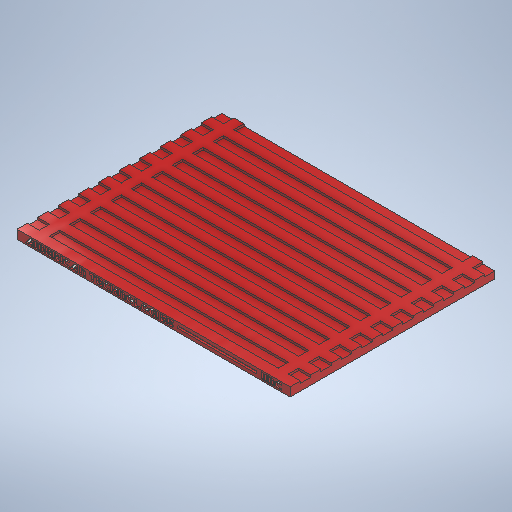
# Autodesk Inventor part: AT-IMC lid
Saved by Autodesk Inventor 2025 (Build 290162000, 162)
## iProperties
Created: 2025-05-10
Part Number: AT-IMC lid
Material: Generic
Document SubType Name: Modeling
Designer: thesn
Density: 1 g/cm^3
Appearance: Default
Author: thesn
Autodesk Inventor part; units mm, degrees
ref_plane "YZ Plane" through (0, 0, 0) normal (1, 0, 0) x (0, 1, 0)
ref_plane "XZ Plane" through (0, 0, 0) normal (0, 1, 0) x (-1, 0, 0)
ref_plane "XY Plane" through (0, 0, 0) normal (0, 0, 1) x (1, 0, 0)
sketch "Sketch1" plane through (0, 0, 0) normal (0, 0, 1) x (1, 0, 0)
  line L0 (0, 0) -> (203.2, 0)
  line L1 (203.2, 0) -> (203.2, 5.08)
  line L2 (203.2, 5.08) -> (0, 5.08)
  line L3 (0, 5.08) -> (0, 0)
  dimension "d0" = 203.2
  dimension "d1" = 5.08
  constraints: 8 end point, 2 parallel, 1 horizontal, 1 perpendicular
  measures "d0" distance of L2.end L1.end
  measures "d1" distance of L1.end L0.end
extrude "Extrusion1" add sketch "Sketch1" along normal blind 152.4
sketch "Sketch2" plane through (0, 0, 0) normal (0, -1, 0) x (1, 0, 0)
  line L0 (5.08, 147.32) -> (198.12, 147.32)
  line L1 (198.12, 147.32) -> (198.12, 5.08)
  line L2 (198.12, 5.08) -> (5.08, 5.08)
  line L3 (5.08, 5.08) -> (5.08, 147.32)
  line L4 (0, 152.4) -> (203.2, 152.4) projected
  line L5 (203.2, 0) -> (203.2, 152.4) projected
  point P0 (0, 0)
  point P1 (101.6, 152.4)
  point P2 (101.6, 147.32)
  point P3 (203.2, 76.2)
  point P4 (198.12, 76.2)
  dimension "d4" = 193.04
  dimension "d5" = 142.24
  dimension "d6" = 0
  dimension "d7" = 0
  constraints: 8 end point, 4 midpoint, 2 parallel, 1 horizontal, 1 perpendicular
  measures "d4" distance of L1.end L2.end
  measures "d5" distance of L0.end L1.end
  measures "d6" horizontal distance of point (101.6, 152.4) point (101.6, 147.32)
  measures "d7" vertical distance of point (203.2, 76.2) point (198.12, 76.2)
extrude "Extrusion2" add sketch "Sketch2" along normal blind 2.54
sketch "Sketch5" plane through (0, 5.08, 0) normal (0, 1, 0) x (1, 0, 0)
  line L0 (0, 0) -> (0, -152.4) projected
  line L1 (203.2, 0) -> (203.2, -152.4) projected
  line L2 (0, -7.62) -> (203.2, -7.62)
  line L3 (203.2, -7.62) -> (203.2, -15.24)
  line L4 (203.2, -15.24) -> (0, -15.24)
  line L5 (0, -15.24) -> (0, -7.62)
  line L6 (203.2, 0) -> (0, 0) projected
  dimension "d21" = 7.62
  dimension "d22" = 7.62
  constraints: 8 end point, 2 parallel, 2 point on line, 1 horizontal, 1 perpendicular
  measures "d21" distance of L2.end L3.end
  measures "d22" distance between parallel lines of L6 L2
extrude "Extrusion5" add sketch "Sketch5" along normal blind 1.524 contours L2 L1 L4 L0
pattern_linear "Rectangular Pattern1" count 10 spacing 15.24 along (0, 0, 1) of "Extrusion5"
sketch "Sketch6" plane through (0, 5.08, 0) normal (0, 1, 0) x (1, 0, 0)
  line L0 (0, 0) -> (203.2, 0) projected
  line L1 (0, -152.4) -> (203.2, -152.4) projected
  line L2 (8.89, 0) -> (16.51, 0)
  line L3 (16.51, 0) -> (16.51, -152.4)
  line L4 (16.51, -152.4) -> (8.89, -152.4)
  line L5 (8.89, -152.4) -> (8.89, 0)
  point P0 (12.7, 0)
  dimension "d28" = 7.62
  dimension "d29" = 12.7
  constraints: 8 end point, 2 parallel, 2 point on line, 1 horizontal, 1 midpoint, 1 perpendicular
  measures "d28" distance of L3.end L4.end
  measures "d29" distance of L0.start point (12.7, 0)
extrude "Extrusion6" add sketch "Sketch6" along normal blind 1.524
pattern_linear "Rectangular Pattern2" count 2 spacing 177.8 along (1, 0, 0) of "Extrusion6"
sketch "Sketch7" plane through (0, 0, 152.4) normal (0, 0, 1) x (1, 0, 0)
  line L0 (6.35, 5.0231) -> (133.882, 5.0231) construction
  line L1 (133.882, 5.0231) -> (133.882, 1.5809) construction
  line L2 (133.882, 1.5809) -> (6.35, 1.5809) construction
  line L3 (6.35, 1.5809) -> (6.35, 5.0231) construction
  line L4 (0, 0) -> (0, 6.604) projected
  line L5 (5.08, 0) -> (5.08, -2.54) projected
  line L6 (174.8972, 4.8148) -> (196.85, 4.8148) construction
  line L7 (196.85, 4.8148) -> (196.85, 1.7892) construction
  line L8 (196.85, 1.7892) -> (174.8972, 1.7892) construction
  line L9 (174.8972, 1.7892) -> (174.8972, 4.8148) construction
  line L10 (203.2, 0) -> (203.2, 6.604) projected
  line L11 (198.12, 0) -> (198.12, -2.54) projected
  line L12 (178.0774, 4.2851) -> (119.6574, 4.2851)
  line L13 (119.6574, 4.2851) -> (119.6574, 2.5071)
  line L14 (119.6574, 2.5071) -> (178.0774, 2.5071)
  line L15 (178.0774, 2.5071) -> (178.0774, 4.2851)
  line L16 (10.6499, 1.9036) -> (10.6499, 1.016)
  line L17 (10.6499, 1.016) -> (12.3003, 1.016)
  line L18 (12.3003, 1.016) -> (12.3003, 5.5835)
  line L19 (12.3003, 5.5835) -> (10.5206, 5.5835)
  spline S0 degree 2 poles (10.5206, 5.5835) (9.9898, 5.5835) (9.2672, 5.2178) (9.0308, 4.8654) knots 0 0 0 1 2 2 2
  line L20 (9.0308, 4.8654) -> (6.3812, 1.016)
  line L21 (6.3812, 1.016) -> (8.3528, 1.016)
  line L22 (8.3528, 1.016) -> (8.9192, 1.9036)
  line L23 (8.9192, 1.9036) -> (10.6499, 1.9036)
  line L24 (9.6775, 3.099) -> (10.409, 4.2454)
  spline S1 degree 2 poles (10.409, 4.2454) (10.4626, 4.3301) (10.5696, 4.3926) (10.6365, 4.3881) knots 0 0 0 1 2 2 2
  line L25 (10.6365, 4.3881) -> (10.6499, 4.3881)
  line L26 (10.6499, 4.3881) -> (10.6499, 3.099)
  line L27 (10.6499, 3.099) -> (9.6775, 3.099)
  line L28 (17.4745, 1.016) -> (17.4745, 4.3881)
  line L29 (17.4745, 4.3881) -> (17.8001, 4.3881)
  spline S2 degree 2 poles (17.8001, 4.3881) (18.1168, 4.3881) (18.429, 4.0134) (18.429, 3.6388) knots 0 0 0 1 2 2 2
  line L30 (18.429, 3.6388) -> (18.429, 1.016)
  line L31 (18.429, 1.016) -> (20.0794, 1.016)
  line L32 (20.0794, 1.016) -> (20.0794, 3.6432)
  spline S3 degree 2 poles (20.0794, 3.6432) (20.0794, 4.6156) (18.9955, 5.5835) (17.9116, 5.5835) knots 0 0 0 1 2 2 2
  line L33 (17.9116, 5.5835) -> (13.2192, 5.5835)
  line L34 (13.2192, 5.5835) -> (13.2192, 1.016)
  line L35 (13.2192, 1.016) -> (14.8695, 1.016)
  line L36 (14.8695, 1.016) -> (14.8695, 4.3881)
  line L37 (14.8695, 4.3881) -> (15.8241, 4.3881)
  line L38 (15.8241, 4.3881) -> (15.8241, 1.016)
  line L39 (15.8241, 1.016) -> (17.4745, 1.016)
  spline S4 degree 2 poles (20.9893, 2.537) (20.9893, 1.7743) (21.8591, 1.016) (22.7378, 1.016) knots 0 0 0 1 2 2 2
  line L40 (22.7378, 1.016) -> (25.6104, 1.016)
  line L41 (25.6104, 1.016) -> (25.6104, 2.2114)
  line L42 (25.6104, 2.2114) -> (23.175, 2.2114)
  spline S5 degree 2 poles (23.175, 2.2114) (22.8895, 2.2114) (22.6352, 2.4344) (22.6397, 2.6485) knots 0 0 0 1 2 2 2
  line L43 (22.6397, 2.6485) -> (22.6397, 2.8314)
  line L44 (22.6397, 2.8314) -> (25.6104, 2.8314)
  line L45 (25.6104, 2.8314) -> (25.6104, 3.8752)
  line L46 (25.6104, 3.8752) -> (22.6397, 3.8752)
  line L47 (22.6397, 3.8752) -> (22.6397, 4.3881)
  line L48 (22.6397, 4.3881) -> (25.6104, 4.3881)
  line L49 (25.6104, 4.3881) -> (25.6104, 5.5835)
  line L50 (25.6104, 5.5835) -> (20.9893, 5.5835)
  line L51 (20.9893, 5.5835) -> (20.9893, 2.537)
  spline S6 degree 2 poles (30.2136, 2.7957) (30.5615, 2.9072) (31.0254, 3.3265) (31.2574, 3.8573) (31.2574, 4.1428) knots 0 0 0 1 2 3 3 3
  spline S7 degree 2 poles (31.2574, 4.1428) (31.2574, 4.513) (30.8827, 5.1643) (30.1244, 5.5746) (29.5579, 5.5835) knots 0 0 0 1 2 3 3 3
  line L52 (29.5579, 5.5835) -> (26.2616, 5.5835)
  line L53 (26.2616, 5.5835) -> (26.2616, 1.016)
  line L54 (26.2616, 1.016) -> (27.912, 1.016)
  line L55 (27.912, 1.016) -> (27.912, 2.6976)
  line L56 (27.912, 2.6976) -> (28.5008, 2.6976)
  line L57 (28.5008, 2.6976) -> (29.2278, 1.694)
  spline S8 degree 2 poles (29.2278, 1.694) (29.4598, 1.3595) (30.1155, 1.016) (30.6641, 1.016) knots 0 0 0 1 2 2 2
  line L58 (30.6641, 1.016) -> (31.4046, 1.016)
  line L59 (31.4046, 1.016) -> (31.4046, 2.2114)
  line L60 (31.4046, 2.2114) -> (30.9541, 2.2114)
  spline S9 degree 2 poles (30.9541, 2.2114) (30.9094, 2.207) (30.6507, 2.2962) (30.508, 2.4434) knots 0 0 0 1 2 2 2
  line L61 (30.508, 2.4434) -> (30.2136, 2.7957)
  spline S10 degree 2 poles (29.2814, 4.3881) (29.433, 4.3837) (29.5936, 4.1919) (29.5936, 4.0625) knots 0 0 0 1 2 2 2
  spline S11 degree 2 poles (29.5936, 4.0625) (29.5936, 3.9332) (29.433, 3.7414) (29.2814, 3.7369) knots 0 0 0 1 2 2 2
  line L62 (29.2814, 3.7369) -> (27.912, 3.7369)
  line L63 (27.912, 3.7369) -> (27.912, 4.3881)
  line L64 (27.912, 4.3881) -> (29.2814, 4.3881)
  line L65 (32.0692, 1.016) -> (33.7196, 1.016)
  line L66 (33.7196, 1.016) -> (33.7196, 5.5835)
  line L67 (33.7196, 5.5835) -> (32.0692, 5.5835)
  line L68 (32.0692, 5.5835) -> (32.0692, 1.016)
  line L69 (36.9579, 1.016) -> (39.0989, 1.016)
  line L70 (39.0989, 1.016) -> (39.0989, 2.2114)
  line L71 (39.0989, 2.2114) -> (37.172, 2.2114)
  spline S12 degree 2 poles (37.172, 2.2114) (36.7928, 2.2159) (36.2888, 2.5281) (36.039, 3.0232) (36.039, 3.2998) knots 0 0 0 1 2 3 3 3
  spline S13 degree 2 poles (36.039, 3.2998) (36.039, 3.5808) (36.2888, 4.0714) (36.7928, 4.3837) (37.172, 4.3881) knots 0 0 0 1 2 3 3 3
  line L72 (37.172, 4.3881) -> (39.0989, 4.3881)
  line L73 (39.0989, 4.3881) -> (39.0989, 5.5835)
  line L74 (39.0989, 5.5835) -> (36.9579, 5.5835)
  spline S14 degree 2 poles (36.9579, 5.5835) (36.097, 5.5746) (34.9506, 4.9189) (34.3752, 3.8841) (34.3752, 3.2998) knots 0 0 0 1 2 3 3 3
  spline S15 degree 2 poles (34.3752, 3.2998) (34.3752, 2.7199) (34.9506, 1.6851) (36.097, 1.0294) (36.9579, 1.016) knots 0 0 0 1 2 3 3 3
  line L75 (43.5951, 1.9036) -> (43.5951, 1.016)
  line L76 (43.5951, 1.016) -> (45.2455, 1.016)
  line L77 (45.2455, 1.016) -> (45.2455, 5.5835)
  line L78 (45.2455, 5.5835) -> (43.4657, 5.5835)
  spline S16 degree 2 poles (43.4657, 5.5835) (42.9349, 5.5835) (42.2123, 5.2178) (41.9759, 4.8654) knots 0 0 0 1 2 2 2
  line L79 (41.9759, 4.8654) -> (39.3264, 1.016)
  line L80 (39.3264, 1.016) -> (41.2979, 1.016)
  line L81 (41.2979, 1.016) -> (41.8644, 1.9036)
  line L82 (41.8644, 1.9036) -> (43.5951, 1.9036)
  line L83 (42.6227, 3.099) -> (43.3542, 4.2454)
  spline S17 degree 2 poles (43.3542, 4.2454) (43.4077, 4.3301) (43.5148, 4.3926) (43.5817, 4.3881) knots 0 0 0 1 2 2 2
  line L84 (43.5817, 4.3881) -> (43.5951, 4.3881)
  line L85 (43.5951, 4.3881) -> (43.5951, 3.099)
  line L86 (43.5951, 3.099) -> (42.6227, 3.099)
  spline S18 degree 2 poles (48.8941, 4.3881) (49.2064, 4.3881) (49.5275, 4.0134) (49.5275, 3.6388) knots 0 0 0 1 2 2 2
  line L87 (49.5275, 3.6388) -> (49.5275, 1.016)
  line L88 (49.5275, 1.016) -> (51.1779, 1.016)
  line L89 (51.1779, 1.016) -> (51.1779, 3.6432)
  spline S19 degree 2 poles (51.1779, 3.6432) (51.1779, 4.6156) (50.094, 5.5835) (49.0101, 5.5835) knots 0 0 0 1 2 2 2
  line L90 (49.0101, 5.5835) -> (46.1643, 5.5835)
  line L91 (46.1643, 5.5835) -> (46.1643, 1.016)
  line L92 (46.1643, 1.016) -> (47.8147, 1.016)
  line L93 (47.8147, 1.016) -> (47.8147, 4.3881)
  line L94 (47.8147, 4.3881) -> (48.8941, 4.3881)
  line L95 (53.5241, 4.3881) -> (55.121, 4.3881)
  line L96 (55.121, 4.3881) -> (55.121, 1.016)
  line L97 (55.121, 1.016) -> (56.7714, 1.016)
  line L98 (56.7714, 1.016) -> (56.7714, 4.3881)
  line L99 (56.7714, 4.3881) -> (58.3682, 4.3881)
  line L100 (58.3682, 4.3881) -> (58.3682, 5.5835)
  line L101 (58.3682, 5.5835) -> (53.542, 5.5835)
  line L102 (53.542, 5.5835) -> (53.5241, 4.3881)
  spline S20 degree 2 poles (59.0239, 2.537) (59.0239, 1.7743) (59.8937, 1.016) (60.7724, 1.016) knots 0 0 0 1 2 2 2
  line L103 (60.7724, 1.016) -> (63.645, 1.016)
  line L104 (63.645, 1.016) -> (63.645, 2.2114)
  line L105 (63.645, 2.2114) -> (61.2095, 2.2114)
  spline S21 degree 2 poles (61.2095, 2.2114) (60.9241, 2.2114) (60.6698, 2.4344) (60.6743, 2.6485) knots 0 0 0 1 2 2 2
  line L106 (60.6743, 2.6485) -> (60.6743, 2.8314)
  line L107 (60.6743, 2.8314) -> (63.645, 2.8314)
  line L108 (63.645, 2.8314) -> (63.645, 3.8752)
  line L109 (63.645, 3.8752) -> (60.6743, 3.8752)
  line L110 (60.6743, 3.8752) -> (60.6743, 4.3881)
  line L111 (60.6743, 4.3881) -> (63.645, 4.3881)
  line L112 (63.645, 4.3881) -> (63.645, 5.5835)
  line L113 (63.645, 5.5835) -> (59.0239, 5.5835)
  line L114 (59.0239, 5.5835) -> (59.0239, 2.537)
  line L115 (66.6201, 1.016) -> (68.7611, 1.016)
  line L116 (68.7611, 1.016) -> (68.7611, 2.2114)
  line L117 (68.7611, 2.2114) -> (66.8342, 2.2114)
  spline S22 degree 2 poles (66.8342, 2.2114) (66.4551, 2.2159) (65.951, 2.5281) (65.7012, 3.0232) (65.7012, 3.2998) knots 0 0 0 1 2 3 3 3
  spline S23 degree 2 poles (65.7012, 3.2998) (65.7012, 3.5808) (65.951, 4.0714) (66.4551, 4.3837) (66.8342, 4.3881) knots 0 0 0 1 2 3 3 3
  line L118 (66.8342, 4.3881) -> (68.7611, 4.3881)
  line L119 (68.7611, 4.3881) -> (68.7611, 5.5835)
  line L120 (68.7611, 5.5835) -> (66.6201, 5.5835)
  spline S24 degree 2 poles (66.6201, 5.5835) (65.7592, 5.5746) (64.6129, 4.9189) (64.0375, 3.8841) (64.0375, 3.2998) knots 0 0 0 1 2 3 3 3
  spline S25 degree 2 poles (64.0375, 3.2998) (64.0375, 2.7199) (64.6129, 1.6851) (65.7592, 1.0294) (66.6201, 1.016) knots 0 0 0 1 2 3 3 3
  line L121 (69.4124, 1.016) -> (71.0628, 1.016)
  line L122 (71.0628, 1.016) -> (71.0628, 2.7021)
  line L123 (71.0628, 2.7021) -> (72.8291, 2.7021)
  line L124 (72.8291, 2.7021) -> (72.8291, 1.016)
  line L125 (72.8291, 1.016) -> (74.4795, 1.016)
  line L126 (74.4795, 1.016) -> (74.4795, 5.5835)
  line L127 (74.4795, 5.5835) -> (72.8291, 5.5835)
  line L128 (72.8291, 5.5835) -> (72.8291, 3.9019)
  line L129 (72.8291, 3.9019) -> (71.0628, 3.9019)
  line L130 (71.0628, 3.9019) -> (71.0628, 5.5835)
  line L131 (71.0628, 5.5835) -> (69.4124, 5.5835)
  line L132 (69.4124, 5.5835) -> (69.4124, 1.016)
  spline S26 degree 2 poles (78.1192, 4.3881) (78.4315, 4.3881) (78.7526, 4.0134) (78.7526, 3.6388) knots 0 0 0 1 2 2 2
  line L133 (78.7526, 3.6388) -> (78.7526, 1.016)
  line L134 (78.7526, 1.016) -> (80.403, 1.016)
  line L135 (80.403, 1.016) -> (80.403, 3.6432)
  spline S27 degree 2 poles (80.403, 3.6432) (80.403, 4.6156) (79.3191, 5.5835) (78.2352, 5.5835) knots 0 0 0 1 2 2 2
  line L136 (78.2352, 5.5835) -> (75.3894, 5.5835)
  line L137 (75.3894, 5.5835) -> (75.3894, 1.016)
  line L138 (75.3894, 1.016) -> (77.0398, 1.016)
  line L139 (77.0398, 1.016) -> (77.0398, 4.3881)
  line L140 (77.0398, 4.3881) -> (78.1192, 4.3881)
  line L141 (83.6904, 1.016) -> (83.8064, 1.016)
  spline S28 degree 2 poles (83.8064, 1.016) (84.6806, 1.0294) (85.8537, 1.6851) (86.4425, 2.7199) (86.4425, 3.2998) knots 0 0 0 1 2 3 3 3
  spline S29 degree 2 poles (86.4425, 3.2998) (86.4425, 3.8841) (85.8537, 4.9189) (84.6806, 5.5746) (83.8064, 5.5835) knots 0 0 0 1 2 3 3 3
  line L142 (83.8064, 5.5835) -> (83.6904, 5.5835)
  spline S30 degree 2 poles (83.6904, 5.5835) (82.8117, 5.5746) (81.643, 4.9189) (81.0542, 3.8841) (81.0542, 3.2998) knots 0 0 0 1 2 3 3 3
  spline S31 degree 2 poles (81.0542, 3.2998) (81.0542, 2.7199) (81.643, 1.6851) (82.8117, 1.0294) (83.6904, 1.016) knots 0 0 0 1 2 3 3 3
  spline S32 degree 2 poles (82.718, 3.2998) (82.718, 3.5808) (82.9277, 4.0714) (83.3603, 4.3837) (83.6904, 4.3881) knots 0 0 0 1 2 3 3 3
  line L143 (83.6904, 4.3881) -> (83.8064, 4.3881)
  spline S33 degree 2 poles (83.8064, 4.3881) (84.132, 4.3837) (84.5647, 4.0714) (84.7788, 3.5808) (84.7788, 3.2998) knots 0 0 0 1 2 3 3 3
  spline S34 degree 2 poles (84.7788, 3.2998) (84.7788, 3.0232) (84.5647, 2.5281) (84.132, 2.2159) (83.8064, 2.2114) knots 0 0 0 1 2 3 3 3
  line L144 (83.8064, 2.2114) -> (83.6904, 2.2114)
  spline S35 degree 2 poles (83.6904, 2.2114) (83.3603, 2.2159) (82.9277, 2.5281) (82.718, 3.0232) (82.718, 3.2998) knots 0 0 0 1 2 3 3 3
  spline S36 degree 2 poles (87.0937, 2.537) (87.0937, 1.7743) (87.9635, 1.016) (88.8423, 1.016) knots 0 0 0 1 2 2 2
  line L145 (88.8423, 1.016) -> (91.8754, 1.016)
  line L146 (91.8754, 1.016) -> (91.8754, 2.2114)
  line L147 (91.8754, 2.2114) -> (89.2794, 2.2114)
  spline S37 degree 2 poles (89.2794, 2.2114) (88.9939, 2.2114) (88.7397, 2.488) (88.7441, 2.7601) knots 0 0 0 1 2 2 2
  line L148 (88.7441, 2.7601) -> (88.7441, 5.5835)
  line L149 (88.7441, 5.5835) -> (87.0937, 5.5835)
  line L150 (87.0937, 5.5835) -> (87.0937, 2.537)
  line L151 (94.9085, 1.016) -> (95.0245, 1.016)
  spline S38 degree 2 poles (95.0245, 1.016) (95.8988, 1.0294) (97.0719, 1.6851) (97.6606, 2.7199) (97.6606, 3.2998) knots 0 0 0 1 2 3 3 3
  spline S39 degree 2 poles (97.6606, 3.2998) (97.6606, 3.8841) (97.0719, 4.9189) (95.8988, 5.5746) (95.0245, 5.5835) knots 0 0 0 1 2 3 3 3
  line L152 (95.0245, 5.5835) -> (94.9085, 5.5835)
  spline S40 degree 2 poles (94.9085, 5.5835) (94.0298, 5.5746) (92.8612, 4.9189) (92.2724, 3.8841) (92.2724, 3.2998) knots 0 0 0 1 2 3 3 3
  spline S41 degree 2 poles (92.2724, 3.2998) (92.2724, 2.7199) (92.8612, 1.6851) (94.0298, 1.0294) (94.9085, 1.016) knots 0 0 0 1 2 3 3 3
  spline S42 degree 2 poles (93.9361, 3.2998) (93.9361, 3.5808) (94.1458, 4.0714) (94.5784, 4.3837) (94.9085, 4.3881) knots 0 0 0 1 2 3 3 3
  line L153 (94.9085, 4.3881) -> (95.0245, 4.3881)
  spline S43 degree 2 poles (95.0245, 4.3881) (95.3501, 4.3837) (95.7828, 4.0714) (95.9969, 3.5808) (95.9969, 3.2998) knots 0 0 0 1 2 3 3 3
  spline S44 degree 2 poles (95.9969, 3.2998) (95.9969, 3.0232) (95.7828, 2.5281) (95.3501, 2.2159) (95.0245, 2.2114) knots 0 0 0 1 2 3 3 3
  line L154 (95.0245, 2.2114) -> (94.9085, 2.2114)
  spline S45 degree 2 poles (94.9085, 2.2114) (94.5784, 2.2159) (94.1458, 2.5281) (93.9361, 3.0232) (93.9361, 3.2998) knots 0 0 0 1 2 3 3 3
  line L155 (100.6358, 1.016) -> (103.214, 1.016)
  line L156 (103.214, 1.016) -> (103.214, 3.6789)
  line L157 (103.214, 3.6789) -> (101.5636, 3.6789)
  line L158 (101.5636, 3.6789) -> (101.5636, 2.2114)
  line L159 (101.5636, 2.2114) -> (100.8544, 2.2114)
  spline S46 degree 2 poles (100.8544, 2.2114) (100.4708, 2.2159) (99.9667, 2.5281) (99.7169, 3.0232) (99.7169, 3.2998) knots 0 0 0 1 2 3 3 3
  spline S47 degree 2 poles (99.7169, 3.2998) (99.7169, 3.5808) (99.9667, 4.0714) (100.4708, 4.3837) (100.8544, 4.3881) knots 0 0 0 1 2 3 3 3
  line L160 (100.8544, 4.3881) -> (103.214, 4.3881)
  line L161 (103.214, 4.3881) -> (103.214, 5.5835)
  line L162 (103.214, 5.5835) -> (100.6358, 5.5835)
  spline S48 degree 2 poles (100.6358, 5.5835) (99.7749, 5.5746) (98.6286, 4.9189) (98.0532, 3.8841) (98.0532, 3.2998) knots 0 0 0 1 2 3 3 3
  spline S49 degree 2 poles (98.0532, 3.2998) (98.0532, 2.7199) (98.6286, 1.6851) (99.7749, 1.0294) (100.6358, 1.016) knots 0 0 0 1 2 3 3 3
  line L163 (103.883, 1.016) -> (105.5334, 1.016)
  line L164 (105.5334, 1.016) -> (105.5334, 5.5835)
  line L165 (105.5334, 5.5835) -> (103.883, 5.5835)
  line L166 (103.883, 5.5835) -> (103.883, 1.016)
  spline S50 degree 2 poles (106.4478, 2.537) (106.4478, 1.7743) (107.3176, 1.016) (108.1963, 1.016) knots 0 0 0 1 2 2 2
  line L167 (108.1963, 1.016) -> (111.0689, 1.016)
  line L168 (111.0689, 1.016) -> (111.0689, 2.2114)
  line L169 (111.0689, 2.2114) -> (108.6334, 2.2114)
  spline S51 degree 2 poles (108.6334, 2.2114) (108.348, 2.2114) (108.0937, 2.4344) (108.0982, 2.6485) knots 0 0 0 1 2 2 2
  line L170 (108.0982, 2.6485) -> (108.0982, 2.8314)
  line L171 (108.0982, 2.8314) -> (111.0689, 2.8314)
  line L172 (111.0689, 2.8314) -> (111.0689, 3.8752)
  line L173 (111.0689, 3.8752) -> (108.0982, 3.8752)
  line L174 (108.0982, 3.8752) -> (108.0982, 4.3881)
  line L175 (108.0982, 4.3881) -> (111.0689, 4.3881)
  line L176 (111.0689, 4.3881) -> (111.0689, 5.5835)
  line L177 (111.0689, 5.5835) -> (106.4478, 5.5835)
  line L178 (106.4478, 5.5835) -> (106.4478, 2.537)
  line L179 (113.0003, 2.8136) -> (114.3206, 2.8136)
  spline S52 degree 2 poles (114.3206, 2.8136) (114.4722, 2.8091) (114.6328, 2.6307) (114.6328, 2.5103) knots 0 0 0 1 2 2 2
  spline S53 degree 2 poles (114.6328, 2.5103) (114.6328, 2.3943) (114.4722, 2.2159) (114.3206, 2.2114) knots 0 0 0 1 2 2 2
  line L180 (114.3206, 2.2114) -> (111.4614, 2.2114)
  line L181 (111.4614, 2.2114) -> (111.4614, 1.016)
  line L182 (111.4614, 1.016) -> (114.7577, 1.016)
  spline S54 degree 2 poles (114.7577, 1.016) (115.2706, 1.0249) (115.9531, 1.4174) (116.2966, 2.0464) (116.2966, 2.4077) knots 0 0 0 1 2 3 3 3
  spline S55 degree 2 poles (116.2966, 2.4077) (116.2966, 2.7601) (115.9531, 3.389) (115.2706, 3.786) (114.7577, 3.7904) knots 0 0 0 1 2 3 3 3
  line L183 (114.7577, 3.7904) -> (113.4374, 3.7904)
  spline S56 degree 2 poles (113.4374, 3.7904) (113.2857, 3.7949) (113.1252, 3.9733) (113.1252, 4.0937) knots 0 0 0 1 2 2 2
  spline S57 degree 2 poles (113.1252, 4.0937) (113.1252, 4.2097) (113.2857, 4.3881) (113.4374, 4.3926) knots 0 0 0 1 2 2 2
  line L184 (113.4374, 4.3926) -> (116.2966, 4.3926)
  line L185 (116.2966, 4.3926) -> (116.2966, 5.588)
  line L186 (116.2966, 5.588) -> (113.0003, 5.588)
  spline S58 degree 2 poles (113.0003, 5.588) (112.4873, 5.5791) (111.8049, 5.1866) (111.4614, 4.5576) (111.4614, 4.2052) knots 0 0 0 1 2 3 3 3
  spline S59 degree 2 poles (111.4614, 4.2052) (111.4614, 3.8484) (111.8049, 3.215) (112.4873, 2.818) (113.0003, 2.8136) knots 0 0 0 1 2 3 3 3
  line L187 (181.8538, 1.016) -> (183.5042, 1.016)
  line L188 (183.5042, 1.016) -> (183.5042, 5.5835)
  line L189 (183.5042, 5.5835) -> (181.8538, 5.5835)
  line L190 (181.8538, 5.5835) -> (181.8538, 1.016)
  line L191 (188.6739, 1.016) -> (188.6739, 4.3881)
  line L192 (188.6739, 4.3881) -> (188.9995, 4.3881)
  spline S60 degree 2 poles (188.9995, 4.3881) (189.3162, 4.3881) (189.6285, 4.0134) (189.6285, 3.6388) knots 0 0 0 1 2 2 2
  line L193 (189.6285, 3.6388) -> (189.6285, 1.016)
  line L194 (189.6285, 1.016) -> (191.2789, 1.016)
  line L195 (191.2789, 1.016) -> (191.2789, 3.6432)
  spline S61 degree 2 poles (191.2789, 3.6432) (191.2789, 4.6156) (190.195, 5.5835) (189.1111, 5.5835) knots 0 0 0 1 2 2 2
  line L196 (189.1111, 5.5835) -> (184.4186, 5.5835)
  line L197 (184.4186, 5.5835) -> (184.4186, 1.016)
  line L198 (184.4186, 1.016) -> (186.069, 1.016)
  line L199 (186.069, 1.016) -> (186.069, 4.3881)
  line L200 (186.069, 4.3881) -> (187.0235, 4.3881)
  line L201 (187.0235, 4.3881) -> (187.0235, 1.016)
  line L202 (187.0235, 1.016) -> (188.6739, 1.016)
  line L203 (194.5127, 1.016) -> (196.6537, 1.016)
  line L204 (196.6537, 1.016) -> (196.6537, 2.2114)
  line L205 (196.6537, 2.2114) -> (194.7268, 2.2114)
  spline S62 degree 2 poles (194.7268, 2.2114) (194.3477, 2.2159) (193.8436, 2.5281) (193.5938, 3.0232) (193.5938, 3.2998) knots 0 0 0 1 2 3 3 3
  spline S63 degree 2 poles (193.5938, 3.2998) (193.5938, 3.5808) (193.8436, 4.0714) (194.3477, 4.3837) (194.7268, 4.3881) knots 0 0 0 1 2 3 3 3
  line L206 (194.7268, 4.3881) -> (196.6537, 4.3881)
  line L207 (196.6537, 4.3881) -> (196.6537, 5.5835)
  line L208 (196.6537, 5.5835) -> (194.5127, 5.5835)
  spline S64 degree 2 poles (194.5127, 5.5835) (193.6518, 5.5746) (192.5055, 4.9189) (191.9301, 3.8841) (191.9301, 3.2998) knots 0 0 0 1 2 3 3 3
  spline S65 degree 2 poles (191.9301, 3.2998) (191.9301, 2.7199) (192.5055, 1.6851) (193.6518, 1.0294) (194.5127, 1.016) knots 0 0 0 1 2 3 3 3
  point P0 (0, 3.302)
  point P1 (6.35, 3.302)
  point P2 (174.8972, 3.302)
  point P3 (203.2, 3.302)
  point P4 (196.85, 3.302)
  point P5 (198.12, -1.27)
  dimension "d35" = 0
  dimension "d36" = 1.27
  dimension "d37" = 0
  dimension "d38" = 1.27
  dimension "d41" = 58.42
  dimension "d42" = 1.778
  constraints: 8 end point, 6 midpoint, 2 parallel, 1 horizontal, 1 perpendicular, 4 other
  measures "d35" vertical distance of point (0, 3.302) point (6.35, 3.302)
  measures "d36" distance between parallel lines of L3 L5
  measures "d37" vertical distance of point (203.2, 3.302) point (196.85, 3.302)
  measures "d38" horizontal distance of point (198.12, -1.27) point (196.85, 3.302)
  measures "d41" distance of L14.end L13.end
  measures "d42" distance of L13.end L12.end
extrude "Extrusion7" cut sketch "Sketch7" against normal blind 1.524
body "Solid1"
